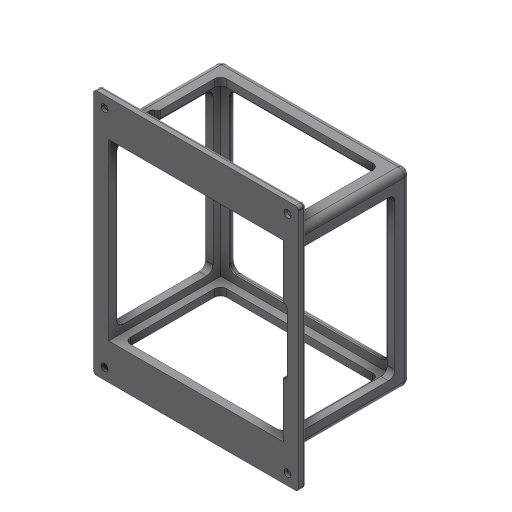
# Autodesk Inventor part: Bauteil3
Saved by Autodesk Inventor 2023 (Build 270158000, 158)
## iProperties
Created: 2025-04-21
Part Number: Bauteil3
Material: Generisch
Document SubType Name: Modeling
Designer: Finn Schröter
Density: 1 g/cm^3
Appearance: Vorgabe
Author: Finn Schröter
Autodesk Inventor part; units mm, degrees
ref_plane "YZ Plane" through (0, 0, 0) normal (1, 0, 0) x (0, 1, 0)
ref_plane "XZ Plane" through (0, 0, 0) normal (0, 1, 0) x (-1, 0, 0)
ref_plane "XY Plane" through (0, 0, 0) normal (0, 0, 1) x (1, 0, 0)
sketch "Skizze1" plane through (0, 0, 0) normal (0, 1, 0) x (-1, 0, 0)
  line L0 (-65, 78.175) -> (65, 78.175)
  line L1 (65, 78.175) -> (65, -78.175)
  line L2 (65, -78.175) -> (-65, -78.175)
  line L3 (-65, -78.175) -> (-65, 78.175)
  line L4 (-65, 78.175) -> (65, -78.175) construction
  line L5 (65, 78.175) -> (-65, -78.175) construction
  point P0 (0, 0)
  dimension "d0" = 156.35
  dimension "d1" = 130
  constraints: 12 end point, 2 midpoint, 2 parallel, 1 horizontal, 1 perpendicular
  measures "d0" distance of L0.end L1.end
  measures "d1" distance of L0.start L0.end
extrude "Extrusion1" add sketch "Skizze1" along normal blind 5
fillet "Rundung1" radius 2 8 edges at (0, 5, -78.175) (65, 5, 0) (-65, 5, 0) (0, 5, 78.175) (-65, 2.5, -78.175) (65, 2.5, -78.175) (-65, 2.5, 78.175) (65, 2.5, 78.175)
sketch "Skizze3" plane through (0, 5, 0) normal (0, 1, 0) x (1, 0, 0)
  line L0 (60, -60) -> (-60, -60)
  line L1 (-60, -60) -> (-60, 60)
  line L2 (-60, 60) -> (60, 60)
  line L3 (60, 60) -> (60, -60)
  line L4 (-63, -78.175) -> (63, -78.175) projected
  line L5 (-91, 0) -> (91, 0) projected
  point P0 (0, 0)
  point P1 (0, -60)
  dimension "d11" = 120
  dimension "d12" = 120
  constraints: 8 end point, 2 parallel, 1 horizontal, 1 midpoint, 1 perpendicular, 1 vertical alignment, 1 other
  measures "d11" distance of L0.start L0.end
  measures "d12" distance of L0.end L1.end
extrude "Extrusion3" add sketch "Skizze3" along normal blind 71
sketch "Skizze4" plane through (0, 0, 0) normal (0, -1, 0) x (1, 0, 0)
  line L0 (55.25, -55.25) -> (-55.25, -55.25)
  line L1 (-55.25, -55.25) -> (-55.25, 55.25)
  line L2 (-55.25, 55.25) -> (55.25, 55.25)
  line L3 (55.25, 55.25) -> (55.25, -55.25)
  line L4 (-91, 0) -> (91, 0) projected
  point P0 (0, 0)
  point P1 (0, -55.25)
  dimension "d17" = 110.5
  dimension "d18" = 110.5
  constraints: 8 end point, 2 parallel, 1 horizontal, 1 midpoint, 1 perpendicular, 1 vertical alignment, 1 other
  measures "d17" distance of L0.start L0.end
  measures "d18" distance of L0.end L1.end
extrude "Extrusion4" cut sketch "Skizze4" against normal blind 71
sketch "Skizze5" plane through (60, 5, -60) normal (0, 0, -1) x (-1, 0, 0)
  line L0 (10, 61) -> (110.5, 61)
  line L1 (110.5, 61) -> (110.5, 0)
  line L2 (110.5, 0) -> (10, 0)
  line L3 (10, 0) -> (10, 61)
  line L4 (120, 0) -> (0, 0) projected
  line L5 (0, 0) -> (0, 71) projected
  line L6 (0, 71) -> (120, 71) projected
  point P0 (60, -5)
  dimension "d21" = 100.5
  dimension "d23" = 10
  dimension "d24" = 10
  dimension "d27" = 61
  constraints: 8 end point, 2 parallel, 1 horizontal, 1 perpendicular
  measures "d21" distance of L0.start L0.end
  measures "d23" distance between parallel lines of L5 L3
  measures "d24" distance between parallel lines of L6 L0
  measures "d27" distance of L2.end L0.start
extrude "Extrusion5" cut sketch "Skizze5" against normal through all
sketch "Skizze6" plane through (60, 5, 60) normal (1, 0, 0) x (0, 0, -1)
  line L0 (10, 61) -> (110.5, 61)
  line L1 (110.5, 61) -> (110.5, 0)
  line L2 (110.5, 0) -> (10, 0)
  line L3 (10, 0) -> (10, 61)
  line L4 (0, 71) -> (120, 71) projected
  line L5 (0, 0) -> (0, 71) projected
  point P0 (60, -5)
  dimension "d28" = 100.5
  dimension "d29" = 61
  dimension "d30" = 10
  dimension "d31" = 10
  constraints: 8 end point, 2 parallel, 1 horizontal, 1 perpendicular
  measures "d28" distance of L0.start L0.end
  measures "d29" distance of L0.end L1.end
  measures "d30" distance between parallel lines of L0 L4
  measures "d31" distance between parallel lines of L5 L3
extrude "Extrusion6" cut sketch "Skizze6" against normal through all
fillet "Rundung2" radius 4 8 edges at (60, 76, 0) (60, 40.5, 60) (0, 76, 60) (-60, 76, 0) (0, 76, -60) (60, 40.5, -60) (-60, 40.5, 60) (-60, 40.5, -60)
sketch "Skizze7" plane through (0, 76, 0) normal (0, 1, 0) x (1, 0, 0)
  line L0 (-50, 50) -> (50, 50)
  line L1 (50, 50) -> (50, -50)
  line L2 (50, -50) -> (-50, -50)
  line L3 (-50, -50) -> (-50, 50)
  point P0 (0, 0)
  point P1 (0, 50)
  point P2 (50, 0)
  dimension "d35" = 100
  dimension "d36" = 100
  constraints: 8 end point, 2 midpoint, 2 parallel, 1 horizontal, 1 horizontal alignment, 1 perpendicular, 1 vertical alignment
  measures "d35" distance of L0.start L0.end
  measures "d36" distance of L0.end L1.end
extrude "Extrusion7" cut sketch "Skizze7" against normal up to next
fillet "Rundung3" radius 4 8 edges at (-50, 73.5, -50) (50, 73.5, -50) (50, 73.5, 50) (-50, 73.5, 50) (-50, 76, 0) (0, 76, 50) (50, 76, 0) (0, 76, -50)
fillet "Rundung4" radius 4 8 edges at (57.625, 66, 50) (50, 66, 57.625) (-57.625, 66, 50) (-50.5, 66, 57.625) (-57.625, 66, -50.5) (-50.5, 66, -57.625) (57.625, 66, -50.5) (50, 66, -57.625)
fillet "Rundung5" radius 4 8 edges at (-57.625, 5, -50.5) (-50.5, 5, -57.625) (-50.5, 5, 57.625) (57.625, 5, -50.5) (-57.625, 5, 50) (50, 5, -57.625) (57.625, 5, 50) (50, 5, 57.625)
fillet "Rundung6" radius 2 20 edges at (48, 5, -60) (53, 5, -60) (60, 5, -53.25) (60, 5, -48.5) (58.8284, 5, -58.8284) (-60, 5, -48.5) (-60, 5, -53.25) (-53.25, 5, -60) (-48.5, 5, -60) (-58.8284, 5, -58.8284) (58.8284, 5, 58.8284) (48, 5, 60) (53, 5, 60) (60, 5, 53) (60, 5, 48) (-58.8284, 5, 58.8284) (-53.25, 5, 60) (-48.5, 5, 60) (-60, 5, 48) (-60, 5, 53)
sketch "Skizze8" plane through (0, 5, 0) normal (0, 1, 0) x (1, 0, 0)
  line L0 (63, 78.175) -> (-63, 78.175) projected
  line L1 (-65, 76.175) -> (-65, -76.175) projected
  line L2 (-63, -78.175) -> (63, -78.175) projected
  line L3 (65, -76.175) -> (65, 76.175) projected
  point P0 (0, 0)
  point P1 (58, -71.175)
  point P2 (-58, -71.175)
  point P3 (-58, 71.175)
  point P4 (58, 71.175)
  dimension "d43" = 7
  dimension "d44" = 7
  dimension "d45" = 7
  dimension "d46" = 7
  constraints: 2 horizontal alignment, 2 vertical alignment
  measures "d43" distance from line of L0 point (-58, 71.175)
  measures "d44" distance from line of point (-58, 71.175) L1
  measures "d45" distance from line of L2 point (58, -71.175)
  measures "d46" distance from line of L3 point (58, -71.175)
hole "Bohrung1" at (58, 5, 71.175) at (-58, 5, 71.175) at (-58, 5, -71.175) at (58, 5, -71.175) direction (0, -1, 0) diameter 4.5 end through all counterbore diameter 8 counterbore depth 3.1
sketch "Skizze9" plane through (-56, 72, 60) normal (0, 0, 1) x (1, 0, 0)
  line L0 (5.5, -46) -> (2.5, -46)
  line L1 (2.5, -46) -> (2.5, -53)
  line L2 (2.5, -53) -> (5.5, -53)
  line L3 (5.5, -53) -> (5.5, -46)
  line L4 (-7, -72) -> (119, -72) projected
  point P0 (56, -72)
  point P1 (5.5, -49.5)
  point P2 (5.5, -63)
  dimension "d54" = 3
  dimension "d55" = 7
  dimension "d56" = 19
  constraints: 8 end point, 2 parallel, 1 horizontal, 1 midpoint, 1 perpendicular, 1 vertical alignment
  measures "d54" distance of L1.end L2.end
  measures "d55" distance of L0.end L1.end
  measures "d56" distance between parallel lines of L2 L4
extrude "Extrusion8" cut sketch "Skizze9" against normal blind 10
fillet "Rundung7" radius 2 2 edges at (-53.5, 19, 57.625) (-53.5, 26, 57.625)
fillet "Rundung8" radius 2 2 edges at (-50.5, 26, 57.625) (-50.5, 19, 57.625)
sketch "Skizze10" plane through (0, 0, 0) normal (0, -1, 0) x (1, 0, 0)
  line L0 (57.75, 20.75) -> (55.25, 20.75)
  line L1 (55.25, 20.75) -> (55.25, -20.25)
  line L2 (55.25, -20.25) -> (57.75, -20.25)
  line L3 (57.75, -20.25) -> (57.75, 20.75)
  line L4 (-55.25, 55.25) -> (55.25, 55.25) projected
  line L5 (55.25, 55.25) -> (55.25, -55.25) projected
  point P0 (0, 0)
  point P1 (56.5, 20.75)
  point P2 (55.25, 0.25)
  point P3 (55.25, 0)
  dimension "d61" = 2.5
  dimension "d62" = 41
  dimension "d63" = 34.5
  constraints: 8 end point, 3 midpoint, 2 parallel, 1 horizontal, 1 perpendicular, 1 vertical alignment
  measures "d61" distance of L1.end L2.end
  measures "d62" distance of L2.end L0.start
  measures "d63" distance from line of L4 point (56.5, 20.75)
extrude "Extrusion9" cut sketch "Skizze10" against normal blind 10
fillet "Rundung9" radius 2 2 edges at (57.75, 2.5, -20.25) (57.75, 2.5, 20.75)
